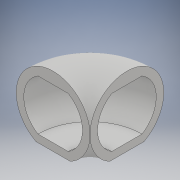
# Autodesk Inventor part: corridor turn
Saved by Autodesk Inventor 2017 (Build 210142000, 142)
## iProperties
Created: 2018-03-04
Part Number: corridor turn
Material: Generic
Document SubType Name: Modeling
Designer: Braxton
Density: 1 g/cm^3
Appearance: Default
Author: Braxton
Autodesk Inventor part; units mm, degrees
ref_plane "YZ Plane" through (0, 0, 0) normal (1, 0, 0) x (0, 1, 0)
ref_plane "XZ Plane" through (0, 0, 0) normal (0, 1, 0) x (-1, 0, 0)
ref_plane "XY Plane" through (0, 0, 0) normal (0, 0, 1) x (1, 0, 0)
sketch "Sketch1" plane through (0, 0, 0) normal (1, 0, 0) x (0, 1, 0)
  line L0 (84.6667, 50.8) -> (84.6667, -50.8)
  line L1 (-84.6667, 50.8) -> (-84.6667, -50.8)
  arc A0 (-110.0667, -57.4059) -> (-110.0667, 57.4059) centre (0, 0) ccw
  arc A1 (84.6667, 50.8) -> (-84.6667, 50.8) centre (0, 0) ccw
  arc A2 (-84.6667, -50.8) -> (84.6667, -50.8) centre (0, 0) ccw
  line L2 (130.9567, -124.1375) -> (-138.9472, -124.1375) construction
  line L3 (-110.0667, -57.4059) -> (-110.0667, 57.4059)
  dimension "d0" = 169.3333
  dimension "d1" = 101.6
  dimension "d11" = 25.4
  constraints: 8 end point, 6 point on circle, 3 centre point, 2 coincident, 2 vertical, 1 horizontal, 1 parallel
  measures "d0" distance between parallel lines of L1 L0
  measures "d1" distance of L0.start L0.end
  measures "d11" distance between parallel lines of L3 L1
revolve "corridor" add sketch "Sketch1" angle 90 about axis through (0, 130.9567, -124.1375) along (0, 1, 0)
body "Solid1"
